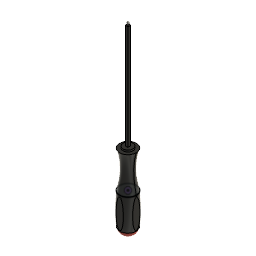
screwdriver (Autodesk Fusion 360 design; units mm, degrees)
part number: 2026-02-05-16-24-56-208
Autodesk Fusion 360 part; units mm, degrees
sketch "Sketch1" plane through (0, 0, 0) normal (0, 1, 0) x (1, 0, 0)
  line L0 (0, 0) -> (0, -40)
  line L1 (3, -40) -> (5, -40)
  spline S0 degree 5 poles (5, -40) (4.8898, -39.6771) (4.6795, -39.0206) (4.3941, -38.0039) (4.0743, -36.5842) (3.7762, -34.7068) (3.5797, -32.7422) (3.4825, -30.7227) (3.4787, -28.7068) (3.5577, -26.7789) (3.7062, -25.0184) (3.9084, -23.4704) (4.1477, -22.1201) (4.4077, -20.8524) (4.672, -19.4794) (4.9242, -17.8124) (5.1478, -15.713) (5.3256, -13.169) (5.4401, -10.2867) (5.475, -7.2403) (5.4152, -4.2365) (5.2821, -2.0261) (5.1306, -0.5447) (5.0062, 0.3559) (4.9381, 0.7844) knots 0 0 0 0 0 0 0.05 0.1 0.15 0.2 0.25 0.3 0.35 0.4 0.45 0.5 0.55 0.6 0.65 0.7 0.75 0.8 0.85 0.9 0.95 1 1 1 1 1 1
  line L2 (0, 0) -> (5, 0) construction
  line L3 (5.456, -2.4762) -> (4.4201, 4.045)
  line L4 (3, -40) -> (3, -41)
  line L5 (3, -41) -> (0, -41)
  line L6 (0, -41) -> (0, -40)
  arc A0 (5, 0) -> (0, 5) centre (0, 0) ccw
  line L7 (0, 0) -> (0, 5)
  line L8 (0, -41) -> (0, -105) construction
  line L9 (0, -105.75) -> (0, -105)
  line L10 (0, -105) -> (0.75, -105)
  line L11 (0, -105) -> (0, -104.25)
  arc A1 (0, -105.75) -> (0, -104.25) centre (0, -105) ccw
  line L12 (4, -23) -> (0, -23) construction
  line L13 (5, -17) -> (0, -17) construction
  point P0 (3.519, -31.1582)
  point P1 (4, -23)
  point P2 (5, -17)
  dimension "d6" = 40
  dimension "d7" = 5
  dimension "d8" = 5
  dimension "d9" = 3
  dimension "d10" = 1
  dimension "d16" = 64
  dimension "d18" = 0.75
  dimension "d22" = 1.5
  dimension "d44" = 4
  dimension "d46" = 5
  constraint coincident L0.start L2.start
  constraint vertical L0
  constraint perpendicular L0 L1
  constraint perpendicular L0 L2
  constraint midpoint S0.end L3
  constraint tangent L3 A0
  constraint vertical L4
  constraint horizontal L5
  constraint vertical L6
  constraint coincident S0.end A0
  constraint perpendicular L2 L7
  constraint perpendicular L5 L8
  constraint coincident L8.end L9.end
  constraint coincident L10.end A1
  constraint perpendicular L9 L10
  constraint coincident L8 L11.end
  constraint parallel L8 L11
  constraint coincident P1 L12.start
  constraint perpendicular L0 L12
  constraint coincident P2 L13.start
  constraint perpendicular L0 L13
  measures "d6" distance of L0.start L0.end
  measures "d7" distance of L0.end L1.end
  measures "d8" distance of L0.start L2.end
  measures "d9" distance of L0.end L1.start
  measures "d10" distance of L0.end L5.end
  measures "d16" distance of L5.end L8.end
  measures "d18" distance of L9.start L8.end
  measures "d22" diameter of A1
  measures "d44" distance of P1 L12.end
  measures "d46" distance of P2 L13.end
revolve "Revolve1" add sketch "Sketch1" angle 360 about axis through (0, 0, 0) along (0, 0, 1) contours L0 L1 S0 L4 L5 L6 A0 L7 makes body 1
sketch "Sketch2" plane through (0, 0, 41) normal (0, 0, 1) x (-1, 0, 0)
  circle A0 centre (0, 0) radius 3
  line L0 (0.75, -0.75) -> (-0.75, -0.75)
  line L1 (-0.75, -0.75) -> (-0.75, 0.75)
  line L2 (-0.75, 0.75) -> (0.75, 0.75)
  line L3 (0.75, 0.75) -> (0.75, -0.75)
  line L4 (0.75, -0.75) -> (-0.75, 0.75) construction
  line L5 (-0.75, -0.75) -> (0.75, 0.75) construction
  line L6 (5, -5) -> (-5, -5)
  line L7 (-5, -5) -> (-5, 5)
  line L8 (-5, 5) -> (5, 5)
  line L9 (5, 5) -> (5, -5)
  line L10 (5, -5) -> (-5, 5) construction
  line L11 (-5, -5) -> (5, 5) construction
  line L12 (5.5, 5.5) -> (-5.5, 5.5)
  line L13 (-5.5, 5.5) -> (-5.5, -5.5)
  line L14 (-5.5, -5.5) -> (5.5, -5.5)
  line L15 (5.5, -5.5) -> (5.5, 5.5)
  line L16 (5.5, 5.5) -> (-5.5, -5.5) construction
  line L17 (-5.5, 5.5) -> (5.5, -5.5) construction
  line L18 (-2.1865, 5.0467) -> (-5.1147, 2.0224)
  line L19 (-5.1147, 2.0224) -> (-5.0467, -2.1865)
  line L20 (-5.0467, -2.1865) -> (-2.0224, -5.1147)
  line L21 (-2.0224, -5.1147) -> (2.1865, -5.0467)
  line L22 (2.1865, -5.0467) -> (5.1147, -2.0224)
  line L23 (5.1147, -2.0224) -> (5.0467, 2.1865)
  line L24 (5.0467, 2.1865) -> (2.0224, 5.1147)
  line L25 (2.0224, 5.1147) -> (-2.1865, 5.0467)
  line L26 (0, -5.5) -> (0, 5.5) construction
  line L27 (5.5, 0) -> (-5.5, 0) construction
  line L28 (2.3106, -5.5372) -> (5.5493, -2.2816)
  line L29 (5.5493, -2.2816) -> (5.5372, 2.3106)
  line L30 (5.5372, 2.3106) -> (2.2816, 5.5493)
  line L31 (2.2816, 5.5493) -> (-2.3106, 5.5372)
  line L32 (-2.3106, 5.5372) -> (-5.5493, 2.2816)
  line L33 (-5.5493, 2.2816) -> (-5.5372, -2.3106)
  line L34 (-5.5372, -2.3106) -> (-2.2816, -5.5493)
  line L35 (-2.2816, -5.5493) -> (2.3106, -5.5372)
  dimension "d12" = 1.5
  dimension "d13" = 1.5
  dimension "d31" = 10
  dimension "d32" = 10
  dimension "d33" = 11
  dimension "d34" = 11
  dimension "d37" = 5.5
  dimension "d38" = 6
  constraint horizontal L0
  constraint perpendicular L0 L1
  constraint parallel L0 L2
  constraint parallel L1 L3
  constraint coincident L4 A0.centre
  constraint coincident L5 A0.centre
  constraint coincident A0.centre origin
  constraint horizontal L6
  constraint perpendicular L6 L7
  constraint parallel L6 L8
  constraint parallel L7 L9
  constraint coincident L10 A0.centre
  constraint coincident L11 A0.centre
  constraint horizontal L12
  constraint perpendicular L12 L13
  constraint parallel L12 L14
  constraint parallel L13 L15
  constraint coincident L16 A0.centre
  constraint coincident L17 A0.centre
  constraint midpoint L14 L26.start
  constraint midpoint L12 L26.end
  constraint midpoint L15 L27.start
  constraint midpoint L13 L27.end
  measures "d12" distance of L1.end L2.end
  measures "d13" distance of L0.end L1.end
  measures "d31" distance of L7.end L8.end
  measures "d32" distance of L6.end L7.end
  measures "d33" distance of L13.end L14.end
  measures "d34" distance of L12.end L13.end
  measures "d37" distance of L18.start A0.centre
  measures "d38" distance of L28.start A0.centre
extrude "Extrude1" add sketch "Sketch2" along normal blind 63.25 contours L0 L1 L2 L3 bodies 1
revolve "Revolve3" add sketch "Sketch1" angle 360 about axis through (0, 0, 105.75) along (0, 0, -1) separate body contours L9 L10 A1 | L10 L11 A1 makes body 2
fillet "Fillet1" radius 0.6 4 edges at (0.75, 0, 104.25) (0, -0.75, 104.25) (-0.75, 0, 104.25) (0, 0.75, 104.25) on bodies 1
sketch "Sketch3" plane through (0, 0, 0) normal (0, 1, 0) x (1, 0, 0)
  point P0 (62, -47)
ref_plane "WorkPlane1" through (6, 0, 0) normal (1, 0, 0) x (0, 1, 0)
sketch "Sketch4" plane through (6, 0, 0) normal (1, 0, 0) x (0, 1, 0)
  line L0 (-2, 40) -> (2, 40)
  line L1 (2, 40) -> (2, -0.5)
  line L2 (2, -0.5) -> (-2, -0.5)
  line L3 (-2, -0.5) -> (-2, 40)
  line L4 (-3, 41) -> (-2.5031, 41) construction
  line L5 (-3, 40) -> (3, 40) construction
  point P0 (0, 40)
  dimension "d27" = 40.5
  dimension "d28" = 4
  constraint horizontal L0
  constraint vertical L1
  constraint horizontal L2
  constraint vertical L3
  constraint perpendicular L1 L4
  constraint perpendicular L1 L5
  constraint midpoint L0 P0
  measures "d27" distance of L0 L2
  measures "d28" distance of L1 L3
extrude "Extrude3" cut sketch "Sketch2" against normal blind 45 contours L6 L9 L14 L15 L28 | L6 L14 L20 L21 L22 L28 L34 | L9 L15 L22 L23 L24 L28 L30 | L6 L20 L21 L22 | L9 L22 L23 L24 | L6 L7 L13 L14 L34 | L8 L9 L12 L15 L30 | L7 L18 L19 L20 | L7 L13 L18 L19 L20 L32 L34 | L8 L12 L18 L24 L25 L30 L32 | L8 L18 L24 L25 | L7 L8 L12 L13 L32 bodies 1
sketch "Sketch5" plane through (0, 0, 41) normal (0, 0, 1) x (-1, 0, 0)
  line L0 (4.5224, -1.809) -> (4.4769, 1.9187)
  line L1 (4.4769, 1.9187) -> (1.809, 4.5224)
  line L2 (1.809, 4.5224) -> (-1.9187, 4.4769)
  line L3 (-1.9187, 4.4769) -> (-4.5224, 1.809)
  line L4 (-4.5224, 1.809) -> (-4.4769, -1.9187)
  line L5 (-4.4769, -1.9187) -> (-1.809, -4.5224)
  line L6 (-1.809, -4.5224) -> (1.9187, -4.4769)
  line L7 (1.9187, -4.4769) -> (4.5224, -1.809)
  line L8 (2.344, 5.5232) -> (-2.2481, 5.5629)
  line L9 (-2.2481, 5.5629) -> (-5.5232, 2.344)
  line L10 (-5.5232, 2.344) -> (-5.5629, -2.2481)
  line L11 (-5.5629, -2.2481) -> (-2.344, -5.5232)
  line L12 (-2.344, -5.5232) -> (2.2481, -5.5629)
  line L13 (2.2481, -5.5629) -> (5.5232, -2.344)
  line L14 (5.5232, -2.344) -> (5.5629, 2.2481)
  line L15 (5.5629, 2.2481) -> (2.344, 5.5232)
  dimension "d39" = 6
  dimension "d42" = 9
  measures "d39" distance of L8.start origin
  measures "d42" distance of L1 L5
ref_plane "WorkPlane2" through (0, 0, 23) normal (0, 0, 1) x (1, 0, 0)
sketch "Sketch6" plane through (0, 0, 23) normal (0, 0, 1) x (1, 0, 0)
  circle A0 centre (0, 0) radius 4
  dimension "d45" = 8
  constraint coincident A0.centre origin
  measures "d45" diameter of A0
ref_plane "WorkPlane3" through (0, 0, 18) normal (0, 0, 1) x (1, 0, 0)
sketch "Sketch7" plane through (0, 0, 18) normal (0, 0, 1) x (1, 0, 0)
  circle A0 centre (0, 0) radius 5
  dimension "d49" = 10
  constraint coincident A0.centre origin
  measures "d49" diameter of A0
sketch "Sketch8" plane through (0, 0, 40) normal (0, 0, 1) x (-1, 0, 0)
  arc A0 (-5, 0) -> (0, -5) centre (0, 0) ccw
  arc A1 (0, -5) -> (5, 0) centre (0, 0) ccw
  arc A2 (5, 0) -> (0, 5) centre (0, 0) ccw
  arc A3 (0, 5) -> (-5, 0) centre (0, 0) ccw
  circle A4 centre (0, 0) radius 3
  line L0 (5.0095, 2.075) -> (2.075, 5.0095)
  line L1 (2.075, 5.0095) -> (-2.075, 5.0095)
  line L2 (-2.075, 5.0095) -> (-5.0095, 2.075)
  line L3 (-5.0095, 2.075) -> (-5.0095, -2.075)
  line L4 (-5.0095, -2.075) -> (-2.075, -5.0095)
  line L5 (-2.075, -5.0095) -> (2.075, -5.0095)
  line L6 (2.075, -5.0095) -> (5.0095, -2.075)
  line L7 (5.0095, -2.075) -> (5.0095, 2.075)
  dimension "d50" = 4.15
  constraint coincident A0.centre A1.centre
  measures "d50" distance of L0.start L6.end
sketch "Sketch9" plane through (0, 0, 40) normal (0, 0, 1) x (-1, 0, 0)
  arc A0 (-5, 0) -> (0, -5) centre (0, 0) ccw
  arc A1 (0, -5) -> (5, 0) centre (0, 0) ccw
  arc A2 (5, 0) -> (0, 5) centre (0, 0) ccw
  arc A3 (0, 5) -> (-5, 0) centre (0, 0) ccw
  circle A4 centre (0, 0) radius 3
  line L0 (4.9751, 2.0608) -> (2.0608, 4.9751)
  line L1 (2.0608, 4.9751) -> (-2.0608, 4.9751)
  line L2 (-2.0608, 4.9751) -> (-4.9751, 2.0608)
  line L3 (-4.9751, 2.0608) -> (-4.9751, -2.0608)
  line L4 (-4.9751, -2.0608) -> (-2.0608, -4.9751)
  line L5 (-2.0608, -4.9751) -> (2.0608, -4.9751)
  line L6 (2.0608, -4.9751) -> (4.9751, -2.0608)
  line L7 (4.9751, -2.0608) -> (4.9751, 2.0608)
  line L8 (0, 0) -> (0, 5) construction
  dimension "d51" = 5.385
  constraint coincident A0.centre A1.centre
  constraint coincident A2.end A3.start
  constraint perpendicular L1 L8
  measures "d51" distance of L0.start A0.centre
loft "Loft1" [suppressed]
delete_face "DeleteFace1" [suppressed]
ref_plane "WorkPlane4" through (0, 0, 41) normal (0, 0, 1) x (1, 0, 0)
split "Split1" [suppressed]
equation "length_tip = 64 mm"
equation "base_length = 46 mm"
equation "base_top = 1 mm"
equation "dome_radius = 6 mm"
equation "base_square_length = 10 mm"
equation "d6 = base_length - dome_radius"
equation "d7 = base_square_length / 2"
equation "d8 = base_square_length / 2"
equation "d9 = base_square_length / 2 - 2 mm"
equation "d10 = base_top"
equation "d14 = length_tip - 0.75 mm"
equation "d16 = length_tip"
equation "d27 = base_length - 5.5 mm"
